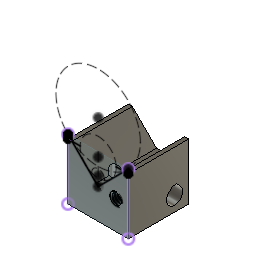
Jig for drilling Conduit (Autodesk Fusion 360 design; units mm, degrees)
Autodesk Fusion 360 part; units mm, degrees
sketch "Base Cube" plane through (0, 0, 0) normal (0, 0, 1) x (1, 0, 0)
  line L0 (0, 0) -> (30, 0)
  line L1 (30, 0) -> (30, -30)
  line L2 (30, -30) -> (0, -30)
  line L3 (0, -30) -> (0, 0)
  dimension "d1" = 30
  dimension "d2" = 30
  constraint horizontal L0
  constraint vertical L1
  constraint horizontal L2
  constraint vertical L3
  constraint coincident L0.start L3.end
  measures "d1" distance of L0.start L0.end
  measures "d2" distance of L0.start L2.end
extrude "Extrude1" add sketch "Base Cube" along normal blind 30
sketch "Front Triangle cut and endstop" plane through (0, -30, 0) normal (0, -1, 0) x (1, 0, 0)
  line L0 (0, 0) -> (30, 0)
  line L1 (30, 0) -> (30, 30)
  line L2 (30, 30) -> (0, 30)
  line L3 (0, 30) -> (0, 0)
  line L4 (0, 30) -> (15, 15)
  line L5 (15, 30) -> (15, 15) construction
  line L6 (30, 30) -> (15, 15)
  circle A0 centre (15, 44.6455) radius 20.964 construction
  circle A1 centre (15, 27.6801) radius 8.9662 construction
  circle A2 centre (15, 19.4901) radius 3.175 construction
  line L7 (14, 16) -> (16, 16)
  line L8 (30, 0) -> (30, 30)
  line L9 (0, 0) -> (0, 30)
  line L10 (30, 28) -> (28, 28)
  line L11 (27.7443, 28) -> (23.9605, 28)
  line L12 (6.0395, 28) -> (2.2557, 28)
  line L13 (2, 28) -> (0, 28)
  circle A3 centre (24, 14.1005) radius 3.175 construction
  point P0 (30, 30)
  point P1 (0, 30)
  dimension "d5" = 90
  dimension "d23" = 41.9281
  dimension "d24" = 17.9324
  dimension "d25" = 6.35
  dimension "d26" = 1
  dimension "d28" = 2
  dimension "d31" = 6.35
  dimension "d39" = 7
  dimension "d40" = 6
  constraint coincident P1 L2.end
  constraint midpoint L2 L5.start
  constraint perpendicular L2 L5
  constraint symmetric P1 L5 P0
  constraint symmetric L4.end L5 L6.end
  constraint coincident A0 P0
  constraint coincident A0 P1
  constraint tangent L6 A1
  constraint tangent L4 A1
  constraint tangent L6 A2
  constraint tangent L4 A2
  constraint coincident L4 L7.start
  constraint coincident L6 L7.end
  constraint horizontal L7
  constraint coincident L8 L10.start
  constraint coincident L9 L13.end
  constraint perpendicular L9 L10
  constraint coincident A1 L11.end
  constraint collinear L10 L12
  constraint coincident L6 L10.end
  constraint coincident A0 L11.start
  constraint collinear L10 L11
  constraint coincident A1 L12.start
  constraint coincident A0 L12.end
  constraint coincident L4 L13.start
  constraint collinear L12 L13
  measures "d5" angle of L4 L6
  measures "d23" diameter of A0
  measures "d24" diameter of A1
  measures "d25" diameter of A2
  measures "d26" distance of L4.end L7
  measures "d28" distance of P0 L10.start
  measures "d31" diameter of A3
  measures "d39" distance of L6 A3.centre
  measures "d40" distance of L8 A3.centre
extrude "Extrude2" cut sketch "Front Triangle cut and endstop" against normal blind 30 contours L2 L4 L6 L7
sketch "Hole for level" plane through (30, 0, 0) normal (1, 0, 0) x (0, 1, 0)
  line L0 (-30, 0) -> (0, 0)
  line L1 (0, 0) -> (0, 30)
  line L2 (0, 30) -> (-30, 30)
  line L3 (-30, 30) -> (-30, 0)
  circle A0 centre (-7, 7) radius 4
  line L4 (-7, 7) -> (-7, 12.6569) construction
  line L5 (-7, 12.6569) -> (-9.8284, 9.8284)
  line L6 (-7, 12.6569) -> (-4.1716, 9.8284)
  line L7 (-6, 11.6569) -> (-8, 11.6569)
  dimension "d8" = 8
  dimension "d9" = 7
  dimension "d10" = 7
  dimension "d27" = 1
  constraint coincident A0.centre L4.start
  constraint vertical L4
  constraint coincident A0 L5.end
  constraint tangent A0 L5
  constraint symmetric L4 L5.end L6.end
  constraint coincident L6 L7.start
  constraint coincident L5 L7.end
  constraint horizontal L7
  constraint perpendicular L5 L6
  measures "d8" diameter of A0
  measures "d9" horizontal distance of L0.end A0.centre
  measures "d10" vertical distance of L0.end A0.centre
  measures "d27" distance of L4.end L7
extrude "Extrude3" cut sketch "Hole for level" against normal blind 30 contours A0 | A0 L5 L6 L7
sketch "Window for level" plane through (0, 0, 0) normal (0, 0, -1) x (1, 0, 0)
  line L0 (30, 30) -> (0, 30) construction
  line L1 (0, 30) -> (0, 0)
  line L2 (0, 0) -> (30, 0)
  line L3 (30, 0) -> (30, 30)
  line L4 (0, 3) -> (0, 11) construction
  line L5 (30, 11) -> (30, 3) construction
  line L6 (0, 11) -> (30, 11) construction
  line L7 (30, 3) -> (0, 3) construction
  line L8 (15, 11) -> (15, 3) construction
  line L9 (10, 4) -> (20, 4)
  arc A0 (20, 4) -> (20, 10) centre (20, 7) ccw
  line L10 (20, 10) -> (10, 10)
  arc A1 (10, 10) -> (10, 4) centre (10, 7) ccw
  line L11 (10, 7) -> (20, 7) construction
  line L12 (30, 4.1716) -> (0, 4.1716)
  line L13 (0, 9.8284) -> (30, 9.8284)
  line L14 (30, 30) -> (0, 30)
  line L15 (15, 30) -> (15, 20.475) construction
  circle A2 centre (15, 20.475) radius 3.175
  point P0 (15, 7)
  point P1 (15, 7)
  dimension "d13" = 1
  dimension "d14" = 3
  dimension "d18" = 6.35
  dimension "d19" = 10
  dimension "d22" = 9.525
  constraint coincident L4.end L6.start
  constraint coincident L5.start L6.end
  constraint coincident L5.end L7.start
  constraint coincident L4.start L7.end
  constraint midpoint L6 L8.start
  constraint midpoint L7 L8.end
  constraint midpoint L8 P1
  constraint tangent L9 A0
  constraint tangent A0 L10
  constraint parallel L9 L10
  constraint tangent L10 A1
  constraint tangent L9 A1
  constraint perpendicular L8 L11
  constraint coincident P1 P0
  constraint midpoint L11 P1
  constraint midpoint L14 L15.start
  constraint perpendicular L14 L15
  constraint coincident L15.end A2.centre
  measures "d13" distance of L6 L10
  measures "d14" radius of A1
  measures "d18" diameter of A2
  measures "d19" distance of A1.centre A0.centre
  measures "d22" distance of L15.start L15.end
extrude "Extrude4" cut sketch "Window for level" against normal blind 4.354 contours A0 A1 L12 L13 | A0 L10 A1 L13 | L9 A0 A1 L12
extrude "Extrude5" cut sketch "Window for level" against normal blind 27.861 contours A2
extrude "Extrude6" cut sketch "Front Triangle cut and endstop" against normal blind 30 contours L3 L4 L9 L13 | L1 L6 L8 L10
hole "Hole1" at (24, -30, 14.1005) direction (0, 1, 0) diameter 5.118 depth 13 tip angle 118
thread "Thread1" "ANSI Unified Screw Threads 0.25 1/4-20 UNC 1B" major diameter 6.35 minor diameter 5.1181 pitch 1.27 angle 60 modelled right hand crest width 0.3461 on face at (24.1276, -25.6667, 11.5447) crest through (24, -29.6825, 11.5415)
equation "d10 = d9"
named bodies: "Jig for drilling Pins"
